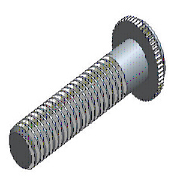
# Autodesk Inventor part: CHA-440-8
Saved by Autodesk Inventor 2018 (Build 220112000, 112)
## iProperties
Created: 2017-02-09
Part Number: CHA-440-8
Material: Aluminium 6061
Catalog Web Link: www.pemnet.com
Description: PEM Śruby dwustronne z ukrytym łbem CHA,CFHA,CHC,CFHC - Calowy
Vendor: PennEngineering®
Document SubType Name: Modeling
Standard: PEM
Designer: Dawid
Manufacturer: PennEngineering®
Language: pl-PL
Size Designation: CHA-440-8
Categories: <MemberInstance><Categories><Category DisplayName="Blacha" InternalName="21944ee9-ad4d-44c9-9b1e-873eb7935d2a" Mnemonic="PEM"><Category DisplayName="Śruby dwustronne" InternalName="a2188e1b-484b-4305-8bf4-ec5c89769453" Mnemonic="pemStuds"><CategoryParameter DisplayName="Oznaczenie serii gwintów" InternalName="03190524-7752-4605-8d0f-16dbfc9a5486" Mnemonic="thrserdsgn"/><CategoryParameter DisplayName="Średnica wałka" InternalName="0798fc74-c739-4cf2-a250-69b5137ecf0b" Mnemonic="grpdia"/><CategoryParameter DisplayName="Gwintów na jednostkę" InternalName="18c8b170-0f21-485b-b6b0-effffc919500" Mnemonic="thrperunit1"/><CategoryParameter DisplayName="Długość nominalna" InternalName="2b53957e-0aee-43be-b71a-49b2debece46" Mnemonic="nomlen"/><CategoryParameter DisplayName="Średnica otworu" InternalName="35967fbd-b0ea-4bd0-85e9-351650fbe2ab" Mnemonic="SMBHD"/><CategoryParameter DisplayName="Długość trzonka" InternalName="4f3018fe-66ab-43a1-8110-181b2668c0c7" Mnemonic="shnklen"/><CategoryParameter DisplayName="Oznaczenie gwintu" InternalName="5793e1d1-8c6a-4152-86f4-a921fb5aab9e" Mnemonic="thrdesign"/><CategoryParameter DisplayName="Minimalna grubość blachy" InternalName="5b7d4485-c0aa-4517-a946-c6a5a269b27c" Mnemonic="SMBMIST"/><CategoryParameter DisplayName="Długość gwintu" InternalName="6caf2edf-e86f-4e63-80ff-b45250d5ceee" Mnemonic="thrlen"/><CategoryParameter DisplayName="Klasa gwintu" InternalName="91059bbb-7712-419d-8465-db77f0d91a13" Mnemonic="thrclss"/><CategoryParameter DisplayName="Typ gwintu" InternalName="a3715b49-09e1-4797-90ad-cbfe5ea9b6ea" Mnemonic="thrtype"/><CategoryParameter DisplayName="Długość uchwytu" InternalName="a513e428-3fb5-4a90-abdd-be9a7d5dab44" Mnemonic="grplen"/><CategoryParameter DisplayName="Średnica nominalna" InternalName="ca11677f-f1e9-4208-b7dc-003eed8d1536" Mnemonic="nomdia"/><Category DisplayName="Ukryty łeb" InternalName="6bb611b0-8967-4548-b4e4-4e1ce6355984" Mnemonic="pemConHeadStuds"/></Category></Category><Category DisplayName="TypDanych" InternalName="23b78d0f-2648-40c6-8793-ca6db495c9e8" Mnemonic="DATATYPE"><CategoryParameter DisplayName="NazwaWyświetlana" InternalName="05415f3d-3907-474b-a020-eb9d644f4cf3" Mnemonic="DISPLAYNAME"/><CategoryParameter DisplayName="Standardowe" InternalName="0c0a119c-1e12-4c84-803f-101930972f5e" Mnemonic="STANDARD"/><CategoryParameter DisplayName="Opis" InternalName="13903e3d-64b1-4950-80da-f627842ea37f" Mnemonic="DESCRIPTION"/><CategoryParameter DisplayName="Oznaczenie" InternalName="2675968c-4ce5-49e0-a4f5-552d29089031" Mnemonic="DESIGNATION"/><CategoryParameter DisplayName="Wiersz domyślny" InternalName="2af9ec52-faaa-4026-b378-f9fa4afca842" Mnemonic="DEFAULTROW"/><CategoryParameter DisplayName="Nazwa folderu" InternalName="3f06958e-8713-4116-9be7-ed6184ecc97b" Mnemonic="FOLDERNAME"/><CategoryParameter DisplayName="Wskazówki do poprawek" InternalName="45a75005-10b1-4dfc-8d6d-dfe629f0b93c" Mnemonic="REVISIONGUID"/><CategoryParameter DisplayName="Nazwa pliku" InternalName="8b46a4cc-9585-4fed-90c3-899f57e09a73" Mnemonic="FILENAME"/><CategoryParameter DisplayName="OrgStd" InternalName="8f5914e1-4693-403f-8ab5-d37768198c9d" Mnemonic="STDSORG"/><CategoryParameter DisplayName="Wersja rodziny" InternalName="914462f6-6e19-4b14-ba84-155b9680b1d0" Mnemonic="FAMILYREVISION"/><CategoryParameter DisplayName="Poprawka standardowa" InternalName="91d5a463-65c2-4fde-b823-3b7fea5e8e17" Mnemonic="STANDARDREVISION"/><CategoryParameter DisplayName="Zmiana elementu" InternalName="a65d44b9-392f-4f4f-857b-e4b3d54996fe" Mnemonic="MEMBERREVISION"/><CategoryParameter DisplayName="FormatKlipu" InternalName="bc51e27b-3422-4e78-93ef-cec197ddf230" Mnemonic="CLIPFORMAT"/><CategoryParameter DisplayName="Producent" InternalName="cd6c7a72-a28a-4e50-99a9-2c7f4e13e5ad" Mnemonic="MANUFACTURER"/><CategoryParameter DisplayName="NazwaWewnętrzna" InternalName="cf1d0246-76d9-4b4a-8305-fa0409afb5c1" Mnemonic="INTERNALNAME"/><CategoryParameter DisplayName="CzyMetryczne" InternalName="e2385c5b-1ea4-4823-96a8-8de651266ec3" Mnemonic="ISMETRIC"/><Category DisplayName="Część" InternalName="c0e0b642-3bcb-4cc8-9e80-f96d35c4afa4" Mnemonic="PART"><CategoryParameter DisplayName="Numer części" InternalName="016b6077-bfbe-49bd-92c9-d8d59c39c941" Mnemonic="PARTNUMBER"/><CategoryParameter DisplayName="Numer katalogowy" InternalName="4dba7c1c-e26c-444e-836c-b08b433409a8" Mnemonic="STOCKNUMBER"/><CategoryParameter DisplayName="Klucz - materiał" InternalName="5c9a8adb-dd2b-4535-b97f-0a94a95fe41f" Mnemonic="MATERIALKEY"/><CategoryParameter DisplayName="Materiał" InternalName="818a152a-d3c3-49ca-80ee-df7d91421b8e" Mnemonic="MATERIAL"/></Category></Category></Categories><FamilyTemplate Id="PEM Concealed-head Studs CHA,CFHA,CHC,CFHC - Inch"><FamilyTemplateParameters><FamilyTemplateParameter ObjectType="kUserParameterObject" ValueType="xs:double" Id="1" ObjectReferenceKey="A_"/><FamilyTemplateParameter ObjectType="kUserParameterObject" ValueType="xs:double" Id="2" ObjectReferenceKey="B_Hole"/><FamilyTemplateParameter ObjectType="kUserParameterObject" ValueType="xs:double" Id="3" ObjectReferenceKey="C1"/><FamilyTemplateParameter ObjectType="kUserParameterObject" ValueType="xs:double" Id="4" ObjectReferenceKey="C_"/><FamilyTemplateParameter ObjectType="kUserParameterObject" ValueType="xs:double" Id="5" ObjectReferenceKey="E_"/><FamilyTemplateParameter ObjectType="kUserParameterObject" ValueType="xs:double" Id="6" ObjectReferenceKey="L"/><FamilyTemplateParameter ObjectType="kUserParameterObject" ValueType="xs:double" Id="8" ObjectReferenceKey="Max_Hole"/><FamilyTemplateParameter ObjectType="kUserParameterObject" ValueType="xs:double" Id="9" ObjectReferenceKey="Min_Depht"/><FamilyTemplateParameter ObjectType="kUserParameterObject" ValueType="xs:double" Id="10" ObjectReferenceKey="Min_Dist"/><FamilyTemplateParameter ObjectType="kUserParameterObject" ValueType="xs:double" Id="11" ObjectReferenceKey="Min_Thick"/><FamilyTemplateParameter ObjectType="kUserParameterObject" ValueType="xs:double" Id="13" ObjectReferenceKey="Thread"/><FamilyTemplateParameter ObjectType="kPropertyObject" ValueType="xs:string" Id="100" ObjectReferenceKey="{32853F0F-3444-11d1-9E93-0060B03C1CA6}" SubObjectId="52"/><FamilyTemplateParameter ObjectType="kPropertyObject" ValueType="xs:string" Id="105" ObjectReferenceKey="{32853F0F-3444-11d1-9E93-0060B03C1CA6}" SubObjectId="5"/><FamilyTemplateParameter ObjectType="kPartComponentDefinitionObject" ValueType="xs:string" Id="110" SubObjectId="Material"/><FamilyTemplateParameter ObjectType="kThreadFeatureObject" ValueType="xs:structure" Id="300" ObjectReferenceKey="1002000010000000b1090000000000008000000000000000" SubObjectId="ThreadInfo"><FamilyTemplateParameter ObjectType="" ValueType="xs:string" Id="301" SubObjectId="ThreadClass"/><FamilyTemplateParameter ObjectType="" ValueType="xs:string" Id="302" SubObjectId="ThreadDesignation"/><FamilyTemplateParameter ObjectType="" ValueType="xs:string" Id="303" SubObjectId="ThreadType"/><FamilyTemplateParameter ObjectType="" ValueType="xs:string" Id="304" SubObjectId="Pitch"/></FamilyTemplateParameter></FamilyTemplateParameters></FamilyTemplate><CategoryParameterMap><ParamToTemplateMap><ParamToTemplate CategoryParameter="//CategoryParameter[@InternalName='05415f3d-3907-474b-a020-eb9d644f4cf3']" ConstantValue="PEM Concealed-head Studs CHA,CFHA,CHC,CFHC - Inch"/><ParamToTemplate CategoryParameter="//CategoryParameter[@InternalName='0c0a119c-1e12-4c84-803f-101930972f5e']" ConstantValue="PEM"/><ParamToTemplate CategoryParameter="//CategoryParameter[@InternalName='13903e3d-64b1-4950-80da-f627842ea37f']" ConstantValue="PEM Concealed-head Studs CHA,CFHA,CHC,CFHC - Inch"/><ParamToTemplate CategoryParameter="//CategoryParameter[@InternalName='2af9ec52-faaa-4026-b378-f9fa4afca842']" ConstantValue="1"/><ParamToTemplate CategoryParameter="//CategoryParameter[@InternalName='3f06958e-8713-4116-9be7-ed6184ecc97b']" ConstantValue="PEM Concealed-head Studs CHA,CFHA,CHC,CFHC - Inch"/><ParamToTemplate CategoryParameter="//CategoryParameter[@InternalName='45a75005-10b1-4dfc-8d6d-dfe629f0b93c']" ConstantValue="3b909f2e-2890-4e77-b3ca-d20ee903a71c"/><ParamToTemplate CategoryParameter="//CategoryParameter[@InternalName='8f5914e1-4693-403f-8ab5-d37768198c9d']" TemplateParameter="101"/><ParamToTemplate CategoryParameter="//CategoryParameter[@InternalName='914462f6-6e19-4b14-ba84-155b9680b1d0']" ConstantValue="11"/><ParamToTemplate CategoryParameter="//CategoryParameter[@InternalName='91d5a463-65c2-4fde-b823-3b7fea5e8e17']" TemplateParameter="103"/><ParamToTemplate CategoryParameter="//CategoryParameter[@InternalName='bc51e27b-3422-4e78-93ef-cec197ddf230']" ConstantValue="CF_INVENTOR.STDPARTS"/><ParamToTemplate CategoryParameter="//CategoryParameter[@InternalName='cd6c7a72-a28a-4e50-99a9-2c7f4e13e5ad']" ConstantValue="PennEngineering®"/><ParamToTemplate CategoryParameter="//CategoryParameter[@InternalName='cf1d0246-76d9-4b4a-8305-fa0409afb5c1']" ConstantValue="78542291-47e4-45dc-a30a-e80681bca12a"/><ParamToTemplate CategoryParameter="//CategoryParameter[@InternalName='e2385c5b-1ea4-4823-96a8-8de651266ec3']" ConstantValue="false"/><ParamToTemplate CategoryParameter="//CategoryParameter[@InternalName='8b46a4cc-9585-4fed-90c3-899f57e09a73']" ConstantValue="CHA-440-8"/><ParamToTemplate CategoryParameter="//CategoryParameter[@InternalName='a65d44b9-392f-4f4f-857b-e4b3d54996fe']" ConstantValue="c87200e5-5fe2-43d8-a855-d4b6a274c29b"/><ParamToTemplate CategoryParameter="//CategoryParameter[@InternalName='35967fbd-b0ea-4bd0-85e9-351650fbe2ab']" TemplateParameter="2"/><ParamToTemplate CategoryParameter="//CategoryParameter[@InternalName='2675968c-4ce5-49e0-a4f5-552d29089031']" TemplateParameter="100"/><ParamToTemplate CategoryParameter="//CategoryParameter[@InternalName='238ecbaf-3e6c-45dd-aa95-4068c8e0fd02']" TemplateParameter="6"/><ParamToTemplate CategoryParameter="//CategoryParameter[@InternalName='818a152a-d3c3-49ca-80ee-df7d91421b8e']" TemplateParameter="110"/><ParamToTemplate CategoryParameter="//CategoryParameter[@InternalName='5b7d4485-c0aa-4517-a946-c6a5a269b27c']" TemplateParameter="11"/><ParamToTemplate CategoryParameter="//CategoryParameter[@InternalName='016b6077-bfbe-49bd-92c9-d8d59c39c941']" TemplateParameter="105"/><ParamToTemplate CategoryParameter="//CategoryParameter[@InternalName='8bbe3f8e-44cf-40a9-a251-3a6edc8168d6']" TemplateParameter="13"/><ParamToTemplate CategoryParameter="//CategoryParameter[@InternalName='ebc0d23b-2cc6-4d2a-b376-d52aae53bab6']" TemplateParameter="301"/><ParamToTemplate CategoryParameter="//CategoryParameter[@InternalName='586d5e89-370a-4089-914f-0110033585c7']" TemplateParameter="302"/><ParamToTemplate CategoryParameter="//CategoryParameter[@InternalName='b4bbb7bc-d6aa-4c9f-a9a9-4152b9f6fe49']" TemplateParameter="303"/></ParamToTemplateMap></CategoryParameterMap></MemberInstance>
Density: 2.7 g/cm^3
Appearance: Aluminium — płaski
IsCustomPart: 0
Author: Dawid
Autodesk Inventor part; units mm, degrees
ref_plane "YZ Plane" through (0, 0, 0) normal (1, 0, 0) x (0, 1, 0)
ref_plane "XZ Plane" through (0, 0, 0) normal (0, 1, 0) x (-1, 0, 0)
ref_plane "XY Plane" through (0, 0, 0) normal (0, 0, 1) x (1, 0, 0)
sketch "Sketch1" plane through (0, 0, 0) normal (1, 0, 0) x (0, 1, 0)
  line L0 (0, 0) -> (2.1717, 0)
  line L1 (2.1717, 0) -> (2.1717, 0.182)
  line L2 (2.1717, 0.182) -> (1.9897, 0.3641)
  line L3 (1.9897, 0.3641) -> (1.9897, 0.5461)
  line L4 (1.9897, 0.5461) -> (2.6035, 0.5461)
  line L5 (2.6035, 0.5461) -> (2.6035, 1.0922)
  line L6 (2.6035, 1.0922) -> (1.4224, 1.0922)
  line L7 (1.4224, 1.0922) -> (1.4224, 13.7922)
  line L8 (1.4224, 13.7922) -> (0, 13.7922)
  line L9 (0, 13.7922) -> (0, 0)
  dimension "d0" = 4.3434
  dimension "d1" = 1.0922
  dimension "d2" = 0.5461
  dimension "d3" = 5.207
  dimension "d4" = 0.182
  dimension "d5" = 0.182
  dimension "d6" = 12.7
  dimension "d7" = 2.8448
  constraints: 20 end point, 8 parallel, 1 horizontal, 1 perpendicular
  measures "d0" diameter of L1 L9
  measures "d1" distance between parallel lines of L0 L6
  measures "d2" distance of L4.end L5.end
  measures "d3" diameter of L5 L9
  measures "d4" distance of L2.end L3.end
  measures "d5" distance from line of L1 L2.end
  measures "d6" distance between parallel lines of L6 L8
  measures "d7" diameter of L7 L9
revolve "Obrót1" add sketch "Sketch1" angle 360 about axis through (0, 0, 13.7922) along (0, 0, -1)
thread "Gwint1" size "4-40 UNC" class "2A" standard "ANSI Unified Screw Threads" length 12.7 offset 1.5748
chamfer "Faza1" distance 0.3048 angle 45 1 edges at (0, -1.4224, 13.7922)
equation "\"d8\" = L"
equation "\"d10\" = C1"
equation "\"d0\" = C_"
equation "\"d1\" = A_"
equation "\"d2\" = 0.5 * A_"
equation "\"d3\" = E_"
equation "\"d4\" = 0.166667 * A_"
equation "\"d5\" = 0.166667 * A_"
equation "\"d6\" = L"
equation "\"d7\" = Thread"
equation "\"A_\" = 1.0922"
equation "\"C_\" = 4.3434"
equation "\"E_\" = 5.207"
equation "\"L\" = 12.7"
equation "\"Thread\" = 2.8448"
equation "\"C1\" = 0.3048"
equation "\"Min_Thick\" = 1.5748"
equation "\"B_Hole\" = 4.3688"
equation "\"Min_Depht\" = 10.922"
equation "\"Min_Dist\" = 3.9624"
equation "\"Max_Hole\" = 3.429"
body "Solid1"
